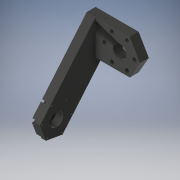
# Autodesk Inventor part: HA07
Saved by Autodesk Inventor 2017 (Build 210142000, 142)
## iProperties
Created: 2018-11-27
Part Number: HA07
Material: ABS Plastic
Document SubType Name: Modeling
Designer: Dell
Density: 1.06 g/cm^3
Appearance: Smooth - Black
Author: Dell
Autodesk Inventor part; units mm, degrees
ref_plane "YZ Plane" through (0, 0, 0) normal (1, 0, 0) x (0, 1, 0)
ref_plane "XZ Plane" through (0, 0, 0) normal (0, 1, 0) x (-1, 0, 0)
ref_plane "XY Plane" through (0, 0, 0) normal (0, 0, 1) x (1, 0, 0)
sketch "Sketch1" plane through (0, 0, 0) normal (0, 0, 1) x (1, 0, 0)
  line L0 (51, 0) -> (25.5, -44.167296) construction
  line L1 (25.5, -44.167296) -> (-25.5, -44.167296) construction
  line L2 (-25.5, -44.167296) -> (-51, 0) construction
  line L3 (-51, 0) -> (-25.5, 44.167296) construction
  line L4 (-25.5, 44.167296) -> (25.5, 44.167296) construction
  line L5 (25.5, 44.167296) -> (51, 0) construction
  circle A0 centre (51, 0) radius 2.5
  circle A1 centre (0, 0) radius 22.5
  circle A2 centre (25.5, 44.167296) radius 2.5
  circle A3 centre (-25.5, 44.167296) radius 2.5
  circle A4 centre (-51, 0) radius 2.5
  circle A5 centre (-25.5, -44.167296) radius 2.5
  circle A6 centre (25.5, -44.167296) radius 2.5
  line L6 (57.5, 0) -> (28.75, -49.796461)
  line L7 (28.75, -49.796461) -> (-28.75, -49.796461)
  line L8 (-28.75, -49.796461) -> (-57.5, 0)
  line L9 (-57.5, 0) -> (-28.75, 49.796461)
  line L10 (-28.75, 49.796461) -> (28.75, 49.796461)
  line L11 (28.75, 49.796461) -> (57.5, 0)
  dimension "d0" = 102
  dimension "d1" = 5
  dimension "d2" = 45
  dimension "d5" = 360
  dimension "d7" = 115
  constraints: 24 end point, 7 centre point, 4 coincident, 2 horizontal alignment, 39 other
  measures "d0" distance of L0.start L2.end
  measures "d1" diameter of A0
  measures "d2" diameter of A1
  measures "d7" distance of L6.start L8.end
extrude "Extrusion1" add sketch "Sketch1" along normal blind 30
sketch "Sketch6" plane through (0, 0, 30) normal (0, 0, 1) x (1, 0, 0)
  line L0 (28.75, 49.796461) -> (-28.75, 49.796461)
  line L1 (-28.75, 49.796461) -> (-111.25, 49.796461)
  line L2 (-111.25, 49.796461) -> (-111.25, -49.796461)
  line L3 (-111.25, -49.796461) -> (-28.75, -49.796461)
  line L4 (-28.75, 49.796461) -> (-57.5, 0)
  line L5 (-57.5, 0) -> (-28.75, -49.796461)
  point P0 (0, 0)
  dimension "d68" = 111.25
  constraints: 6 end point, 2 perpendicular, 1 horizontal
  measures "d68" distance from line of point (0, 0) L2
extrude "Extrusion6" add sketch "Sketch6" against normal blind 30
sketch "Sketch7" plane through (-111.25, -49.796461, 30) normal (-1, 0, 0) x (0, 0, 1)
  line L0 (0, 99.592921) -> (0, 0)
  line L1 (0, 99.592921) -> (-30, 99.592921)
  line L2 (-30, 0) -> (-30, 99.592921)
  line L3 (0, 0) -> (-30, 0)
  line L4 (151.055088, -70.630747) -> (188.015376, -114.678302)
  line L5 (188.015376, -114.678302) -> (168.349218, -168.710628)
  line L6 (168.349218, -168.710628) -> (111.722772, -178.695398)
  line L7 (111.722772, -178.695398) -> (74.762484, -134.647843)
  line L8 (74.762484, -134.647843) -> (94.428642, -80.615517)
  line L9 (94.428642, -80.615517) -> (151.055088, -70.630747)
  line L10 (74.762484, -134.647843) -> (188.015376, -114.678302)
  line L11 (-30, -9.796776) -> (74.762484, -134.647843)
  line L12 (-30, -9.796776) -> (-30, 109.389697)
  line L13 (-30, 109.389697) -> (0, 109.389697)
  line L14 (0, 109.389697) -> (151.055088, -70.630747)
  point P0 (131.38893, -124.663073)
  point P1 (-30, 49.796461)
  dimension "d43" = 115
  dimension "d48" = 40
  dimension "d49" = 235
  constraints: 22 end point, 2 collinear, 2 midpoint, 1 perpendicular, 1 vertical, 1 vertical alignment, 13 other
  measures "d43" distance of L7.end L4.end
  measures "d48" angle of L14 L0
  measures "d49" distance of L13.end L4.start
extrude "Extrusion7" add sketch "Sketch7" against normal blind 30
sketch "Sketch8" plane through (0, 0, 0) normal (0, 0, -1) x (-1, 0, 0)
  line L0 (-68.812342, 0) -> (-34.406171, 59.593237)
  line L1 (-34.406171, 59.593237) -> (34.406171, 59.593237)
  line L2 (34.406171, 59.593237) -> (68.812342, 0)
  line L3 (68.812342, 0) -> (34.406171, -59.593237)
  line L4 (34.406171, -59.593237) -> (-34.406171, -59.593237)
  line L5 (-34.406171, -59.593237) -> (-68.812342, 0)
  line L6 (111.25, 59.593237) -> (81.25, 59.593237)
  line L7 (81.25, 59.593237) -> (34.406171, 59.593237)
  line L8 (81.25, -59.593237) -> (34.406171, -59.593237)
  line L9 (111.25, -59.593237) -> (81.25, -59.593237)
  line L10 (81.25, 49.796461) -> (-28.75, 49.796461)
  line L11 (-28.75, 49.796461) -> (-57.5, 0)
  line L12 (-57.5, 0) -> (-28.75, -49.796461)
  line L13 (-28.75, -49.796461) -> (81.25, -49.796461)
  line L14 (81.25, -59.593237) -> (81.25, -49.796461)
  line L15 (111.25, -59.593237) -> (81.25, -59.593237)
  line L16 (111.25, 59.593237) -> (111.25, -59.593237)
  line L17 (111.25, 59.593237) -> (81.25, 59.593237)
  line L18 (81.25, 49.796461) -> (81.25, 59.593237)
  circle A0 centre (-51, 0) radius 2.5
  circle A1 centre (-25.5, 44.167296) radius 2.5
  circle A2 centre (25.5, 44.167296) radius 2.5
  circle A3 centre (51, 0) radius 2.5
  circle A4 centre (25.5, -44.167296) radius 2.5
  circle A5 centre (-25.5, -44.167296) radius 2.5
  circle A6 centre (0, 0) radius 22.5
  line L19 (81.25, 49.796461) -> (-28.75, 49.796461)
  line L20 (40.062342, 49.796461) -> (-28.75, 49.796461)
  line L21 (-28.75, 49.796461) -> (-57.5, 0)
  line L22 (-28.75, -49.796461) -> (-57.5, 0)
  line L23 (-28.75, -49.796461) -> (-57.5, 0)
  line L24 (-28.75, -49.796461) -> (40.062342, -49.796461)
  line L25 (-28.75, -49.796461) -> (81.25, -49.796461)
  line L26 (34.406171, 59.593237) -> (81.25, 59.593237)
  line L27 (81.25, 59.593237) -> (81.25, -164.474763)
  line L28 (81.25, 49.796461) -> (81.25, 59.593237)
  line L29 (40.062342, 49.796461) -> (81.25, 49.796461)
  line L30 (40.062342, -49.796461) -> (81.25, -49.796461)
  line L31 (81.25, -228.491859) -> (81.25, -59.593237)
  line L32 (81.25, -49.796461) -> (81.25, -59.593237)
  line L33 (81.25, -59.593237) -> (34.406171, -59.593237)
  constraints: 36 end point, 6 collinear, 4 point on line, 2 parallel, 1 coincident, 1 perpendicular, 1 vertical, 13 other
extrude "Extrusion8" add sketch "Sketch8" against normal blind 30 contours L0 L1 L2 L10 L11 L12 L13 L3 L4 L5 | L7 L18 L10 L2 | L3 L13 L14 L8
sketch "Sketch9" plane through (-111.25, -228.491859, 141.722772) normal (-1, 0, 0) x (0, 0.1736482, 0.9848078)
  line L0 (57.5, 0) -> (86.25, 49.796461) construction
  line L1 (0, 0) -> (57.5, 0) construction
  line L2 (57.5, 0) -> (0, 0)
  line L3 (0, 0) -> (-28.75, 49.796461) construction
  line L4 (-28.75, 49.796461) -> (0, 99.592921) construction
  line L5 (0, 99.592921) -> (57.5, 99.592921) construction
  line L6 (57.5, 99.592921) -> (86.25, 49.796461) construction
  line L7 (86.25, 49.796461) -> (57.5, 0)
  circle A0 centre (3.25, 93.963756) radius 2.5
  line L8 (0, 99.592921) -> (28.75, 49.796461) construction
  circle A1 centre (28.75, 49.796461) radius 22.5
  circle A2 centre (-22.25, 49.796461) radius 2.5
  circle A3 centre (3.25, 5.629165) radius 2.5
  circle A4 centre (54.25, 5.629165) radius 2.5
  circle A5 centre (79.75, 49.796461) radius 2.5
  circle A6 centre (54.25, 93.963756) radius 2.5
  point P0 (-99.89249, 249.630455)
  dimension "d52" = 5
  dimension "d53" = 45
  dimension "d55" = 51
  dimension "d58" = 360
  constraints: 14 end point, 7 centre point, 1 coincident, 1 point on line, 26 other
  measures "d52" diameter of A0
  measures "d53" diameter of A1
  measures "d55" distance of L8.end A0.centre
extrude "Extrusion9" cut sketch "Sketch9" against normal through all
ref_plane "Work Plane1" through (0, 0, 15) normal (0, 0, 1) x (1, 0, 0)
sketch "Sketch10" plane through (0, 0, 15) normal (0, 0, 1) x (1, 0, 0)
  circle A0 centre (25.5, 44.167296) radius 2.5
  circle A1 centre (25.5, 44.167296) radius 6.5
  circle A2 centre (-25.5, 44.167296) radius 6.5
  circle A3 centre (-51, 0) radius 6.5
  circle A4 centre (-25.5, -44.167296) radius 6.5
  circle A5 centre (25.5, -44.167296) radius 6.5
  circle A6 centre (51, 0) radius 6.5
  point P0 (0, 0)
  dimension "d70" = 13
  dimension "d73" = 360
  constraints: 6 centre point, 1 coincident, 13 other
  measures "d70" diameter of A1
extrude "Extrusion10" cut sketch "Sketch10" along normal through all contours A0 | A1 | A2 | A3 | A4 | A5 | A6
sketch "Sketch11" plane through (-111.25, 59.593237, 0) normal (-1, 0, 0) x (0, 0, 1)
  circle A0 centre (161.38893, -234.05277) radius 22.5
  point P0 (0, -59.593237)
extrude "Extrusion11" add sketch "Sketch11" against normal blind 5
sketch "Sketch12" plane through (0, 0, 30) normal (0, 0, 1) x (1, 0, 0)
  circle A0 centre (0, 0) radius 22.5 projected
extrude "Extrusion12" add sketch "Sketch12" against normal blind 5
sketch "Sketch14" plane through (-111.25, 59.593237, 0) normal (-1, 0, 0) x (0, 0, 1)
  circle A0 centre (161.38893, -234.05277) radius 22.5 construction
  circle A1 centre (211.614125, -225.196713) radius 2.5 construction
  circle A2 centre (211.614125, -225.196713) radius 2.5
  circle A3 centre (211.614125, -225.196713) radius 6.5
  circle A4 centre (178.831957, -186.128446) radius 6.5
  circle A5 centre (128.606762, -194.984503) radius 6.5
  circle A6 centre (111.163735, -242.908827) radius 6.5
  circle A7 centre (143.945903, -281.977093) radius 6.5
  circle A8 centre (194.171098, -273.121036) radius 6.5
  point P0 (0, -59.593237)
  dimension "d81" = 13
  dimension "d84" = 360
  constraints: 6 centre point, 1 coincident, 13 other
  measures "d81" diameter of A3
extrude "Extrusion13" cut sketch "Sketch14" against normal blind 15 contours A2 | A3 | A4 | A5 | A6 | A7 | A8
sketch "Sketch16" plane through (-81.25, -49.796461, 30) normal (1, 0, 0) x (0, 0, -1)
  circle A0 centre (-131.38893, -124.663073) radius 22.5
  line L0 (-120.488138, -104.980015) -> (0, 64.828282)
  line L1 (-149.738911, -111.642772) -> (0, 99.389697)
  line L2 (0, -9.796776) -> (0, 109.389697)
  circle A1 centre (-131.38893, -124.663073) radius 22.5
  line L3 (0, 49.796461) -> (0, 109.389697)
  line L4 (30, 109.389697) -> (0, 109.389697)
  line L5 (-120.488138, -104.980015) -> (-149.738911, -111.642772)
  line L6 (0, 64.828282) -> (0, 99.389697)
  point P0 (30, 49.796461)
  dimension "d89" = 20
  dimension "d91" = 10
  constraints: 8 end point, 2 point on circle, 2 point on line, 1 collinear, 1 parallel, 1 tangent
  measures "d89" distance between parallel lines of L0 L1
  measures "d91" distance from line of L4 L1.end
extrude "Extrusion14" cut sketch "Sketch16" against normal blind 25 contours A0 L1 L2 L0
sketch "Sketch18" plane through (0, 0, 30) normal (0, 0, 1) x (1, 0, 0)
  circle A0 centre (25.5, -44.167296) radius 6.5
  circle A1 centre (-51, 0) radius 6.5
  circle A2 centre (25.5, 44.167296) radius 6.5
  circle A3 centre (-25.5, 44.167296) radius 6.5
  circle A4 centre (-25.5, -44.167296) radius 6.5
  circle A5 centre (51, 0) radius 6.5
  line L0 (-81.25, -59.593237) -> (-81.25, 15.031821)
  line L1 (-81.25, -59.593237) -> (34.406171, -59.593237)
  line L2 (34.406171, -59.593237) -> (68.812342, 0)
  line L3 (68.812342, 0) -> (34.406171, 59.593237)
  line L4 (34.406171, 59.593237) -> (-81.25, 59.593237)
  line L5 (-81.25, 49.593237) -> (-81.25, 59.593237)
  line L6 (-81.25, 49.593237) -> (-106.25, 49.593237)
  line L7 (-106.25, 49.593237) -> (-106.25, 15.031821)
  line L8 (-81.25, 15.031821) -> (-106.25, 15.031821)
  circle A6 centre (0, 0) radius 22.5
  circle A7 centre (0, 0) radius 22.5
  line L9 (-21.706267, 5.923509) -> (-81.25, 15.031821)
  line L10 (-81.25, -161.439233) -> (-81.25, 49.593237)
  line L11 (-81.25, 49.593237) -> (-2.834809, 22.320705)
  line L12 (-21.706267, 5.923509) -> (-2.834809, 22.320705)
  dimension "d94" = 25
  constraints: 6 end point, 2 point on circle, 2 other
  measures "d94" distance of L9.start L11.end
extrude "Extrusion15" cut sketch "Sketch18" against normal blind 25 contours L10 L11 A6 L9 | L8 L7 L6 L10 | L12 A6 | A6 L12
sketch "Sketch19" plane through (-81.25, -49.796461, 30) normal (1, 0, 0) x (0, 0, -1)
  arc A0 (-149.738911, -111.642772) -> (-120.488138, -104.980015) centre (-131.38893, -124.663073) ccw
  line L0 (0, 64.828282) -> (-120.488138, -104.980015)
  line L1 (-149.738911, -111.642772) -> (0, 99.389697)
  line L2 (0, 49.796461) -> (0, 109.389697)
  line L3 (0, 64.828282) -> (-120.488138, -104.980015)
  line L4 (-149.738911, -111.642772) -> (0, 99.389697)
  arc A1 (-120.488138, -104.980015) -> (-149.738911, -111.642772) centre (-131.38893, -124.663073) ccw
  line L5 (0, 99.389697) -> (25, 99.389697)
  line L6 (0, 64.828282) -> (0, 99.389697)
  point P0 (30, 49.796461)
  constraints: 2 end point, 2 point on circle, 1 centre point, 1 concentric, 1 vertical
extrude "Extrusion16" add sketch "Sketch19" against normal blind 2 contours L1 L2 L0 A1
fillet "Fillet1" radius 15 3 edges at (-106.25, 32.3125, 5) (-106.25, 49.5932, 17.5) (-93.75, 49.5932, 5)
sketch "Sketch20" plane through (-106.25, 59.593237, 0) normal (1, 0, 0) x (0, 0, -1)
  line L0 (-178.899264, -281.529877) -> (-173.833101, -252.798239)
  line L1 (-173.833101, -252.798239) -> (-156.106562, -255.923906)
  line L2 (-156.106562, -255.923906) -> (-161.172725, -284.655544)
  line L3 (-161.172725, -284.655544) -> (-178.899264, -281.529877)
  circle A0 centre (-161.38893, -234.05277) radius 22.5
  line L4 (-164.969832, -254.361072) -> (-161.38893, -234.05277)
  line L5 (-198.349218, -278.100325) -> (-141.722772, -288.085096)
  point P0 (0, -59.593237)
  dimension "d100" = 18
  constraints: 10 end point, 4 perpendicular, 2 point on circle, 2 point on line, 1 midpoint
  measures "d100" distance between parallel lines of L2 L0
extrude "Extrusion17" cut sketch "Sketch20" along normal blind 10 contours L0 A0 L2 L3
sketch "Sketch22" plane through (-111.25, 59.593237, 30) normal (0, 1, 0) x (1, 0, 0)
  line L0 (108.415191, 25) -> (89.543733, 25)
  line L1 (89.543733, 0) -> (89.543733, 25)
  line L2 (108.415191, 0) -> (89.543733, 0)
  line L3 (108.415191, 0) -> (108.415191, 25)
  line L4 (88.75, 30) -> (133.75, 30)
  circle A0 centre (51.25, 15) radius 2.5
  point P0 (111.25, 30)
  dimension "d103" = 5
  dimension "d104" = 15
  dimension "d105" = 60
  constraints: 1 centre point
  measures "d103" diameter of A0
  measures "d104" distance from line of L2 A0.centre
  measures "d105" horizontal distance of A0.centre point (111.25, 30)
extrude "Extrusion18" cut sketch "Sketch22" against normal blind 35 contours A0
body "Solid1"
